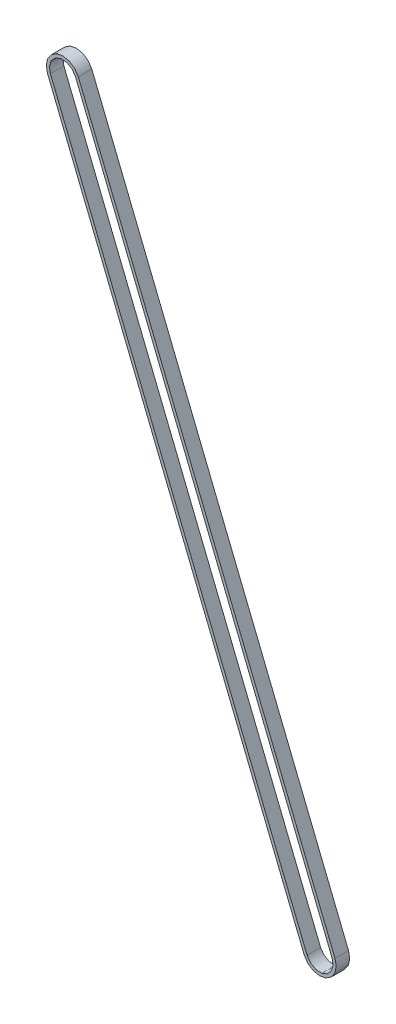
# Autodesk Inventor part: ремень оси y
Saved by Autodesk Inventor 2017 (Build 210142000, 142)
## iProperties
Part Number: ремень оси y
Material: Типовые
Document SubType Name: Modeling
Designer: Max
Mass: 5.47604 g
Surface Area: 96.4825 cm^2
Volume: 5.47604 cm^3
Density: 1 g/cm^3
Appearance: Резина — черная — версия 1.1
Author: Max
Autodesk Inventor part; units mm, degrees
ref_plane "YZ Plane" through (0, 0, 0) normal (1, 0, 0) x (0, 1, 0)
ref_plane "XZ Plane" through (0, 0, 0) normal (0, 1, 0) x (-1, 0, 0)
ref_plane "XY Plane" through (0, 0, 0) normal (0, 0, 1) x (1, 0, 0)
sketch "Эскиз1" plane through (0, 0, 0) normal (0, 0, 1) x (1, 0, 0)
  arc A0 (-5.5627, -2.2486) -> (5.5627, 2.2486) centre (0, 0) ccw
  circle A1 centre (-114.2699, 282.6835) radius 2.5 projected
  arc A2 (-108.7072, 284.9321) -> (-119.8326, 280.4348) centre (-114.2699, 282.6835) ccw
  arc A3 (-107.4093, 285.4568) -> (-121.1306, 279.9102) centre (-114.2699, 282.6835) ccw
  line L0 (-107.4093, 285.4568) -> (6.8607, 2.7733)
  line L1 (-6.8607, -2.7733) -> (-121.1306, 279.9102)
  line L2 (5.5627, 2.2486) -> (-108.7072, 284.9321)
  line L3 (-119.8326, 280.4348) -> (-5.5627, -2.2486)
  arc A4 (-6.8607, -2.7733) -> (6.8607, 2.7733) centre (0, 0) ccw
  dimension "d0" = 12
  dimension "d1" = 1.4
  dimension "d3" = 12
  dimension "d4" = 1.4
  constraints: 8 end point, 8 point on circle, 7 tangent, 4 centre point, 4 coincident, 1 parallel
  measures "d0" diameter of A2
  measures "d1" radial gap between concentric circles of A2 A3
  measures "d3" diameter of A0
  measures "d4" distance between parallel lines of L2 L0
extrude "Выдавливание1" add sketch "Эскиз1" along normal mid plane 6 contours L0 A4 L1 A3
